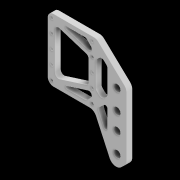
# Autodesk Inventor part: UpperShoulderBracket
Saved by Autodesk Inventor 2020 (Build 240168000, 168)
## iProperties
Created: 2020-04-26
Part Number: UpperShoulderBracket
Material: Generic
Document SubType Name: Sheet Metal
Designer: valer
Density: 1 g/cm^3
Sheet Metal Rule: Default
Appearance: Default
Author: valer
Autodesk Inventor part; units mm, degrees
ref_plane "YZ Plane" through (0, 0, 0) normal (1, 0, 0) x (0, 1, 0)
ref_plane "XZ Plane" through (0, 0, 0) normal (0, 1, 0) x (-1, 0, 0)
ref_plane "XY Plane" through (0, 0, 0) normal (0, 0, 1) x (1, 0, 0)
sketch "Sketch1" plane through (0, 0, 0) normal (0, 0, 1) x (1, 0, 0)
  line L0 (-42.4511, 36.83) -> (-26.4283, 36.83)
  arc A0 (-24.6322, 36.0861) -> (-26.4283, 36.83) centre (-26.4283, 34.29) ccw
  line L1 (-24.6322, 36.0861) -> (-21.0157, 32.4696)
  arc A1 (-23.5785, 28.252) -> (-21.0157, 32.4696) centre (-22.8118, 30.6735) ccw
  line L2 (-23.5785, 28.252) -> (-42.8345, 34.3492)
  arc A2 (-42.4511, 36.83) -> (-42.8345, 34.3492) centre (-42.4511, 35.56) ccw
  line L3 (-42.8345, -8.9492) -> (-23.5785, -2.852)
  arc A3 (-21.0157, -7.0696) -> (-23.5785, -2.852) centre (-22.8118, -5.2735) ccw
  line L4 (-21.0157, -7.0696) -> (-24.6322, -10.6861)
  arc A4 (-26.4283, -11.43) -> (-24.6322, -10.6861) centre (-26.4283, -8.89) ccw
  line L5 (-26.4283, -11.43) -> (-42.4511, -11.43)
  arc A5 (-42.8345, -8.9492) -> (-42.4511, -11.43) centre (-42.4511, -10.16) ccw
  line L6 (-52.9416, -3.8174) -> (-52.9416, 29.2174)
  arc A6 (-48.8082, 32.2443) -> (-52.9416, 29.2174) centre (-49.7666, 29.2174) ccw
  line L7 (-48.8082, 32.2443) -> (-25.2598, 24.7879)
  arc A7 (-23.0433, 21.7611) -> (-25.2598, 24.7879) centre (-26.2183, 21.7611) ccw
  line L8 (-23.0433, 21.7611) -> (-23.0433, 3.6389)
  arc A8 (-25.2598, 0.6121) -> (-23.0433, 3.6389) centre (-26.2183, 3.6389) ccw
  line L9 (-25.2598, 0.6121) -> (-48.8082, -6.8443)
  arc A9 (-52.9416, -3.8174) -> (-48.8082, -6.8443) centre (-49.7666, -3.8174) ccw
  line L10 (-6.35, 22.8627) -> (-6.35, 2.5373)
  arc A10 (-7.3432, 0.2307) -> (-6.35, 2.5373) centre (-9.525, 2.5373) ccw
  line L11 (-7.3432, 0.2307) -> (-9.3482, -1.6658)
  arc A11 (-13.775, -1.6043) -> (-9.3482, -1.6658) centre (-11.53, 0.6408) ccw
  line L12 (-13.775, -1.6043) -> (-15.7633, 0.384)
  arc A12 (-16.6933, 2.629) -> (-15.7633, 0.384) centre (-13.5183, 2.629) ccw
  line L13 (-16.6933, 2.629) -> (-16.6933, 22.771)
  arc A13 (-15.7633, 25.016) -> (-16.6933, 22.771) centre (-13.5183, 22.771) ccw
  line L14 (-15.7633, 25.016) -> (-13.775, 27.0043)
  arc A14 (-9.3482, 27.0658) -> (-13.775, 27.0043) centre (-11.53, 24.7592) ccw
  line L15 (-9.3482, 27.0658) -> (-7.3432, 25.1693)
  arc A15 (-6.35, 22.8627) -> (-7.3432, 25.1693) centre (-9.525, 22.8627) ccw
  circle A16 centre (-55.8683, 24.7103) radius 1.27
  circle A17 centre (-55.8683, 0.7103) radius 1.27
  circle A18 centre (-19.8683, -11.2897) radius 1.27
  circle A19 centre (-19.8683, 12.7103) radius 1.27
  circle A20 centre (-19.8683, 36.7103) radius 1.27
  circle A21 centre (-19.8683, 24.7103) radius 1.27
  circle A22 centre (-19.8683, 0.7103) radius 1.27
  circle A23 centre (-55.8683, -11.2897) radius 1.27
  circle A24 centre (-55.8683, 12.7103) radius 1.27
  circle A25 centre (-55.8683, 36.7103) radius 1.27
  arc A26 (-54.2116, 40.64) -> (-59.2916, 35.56) centre (-54.2116, 35.56) ccw
  line L16 (-59.2916, -10.16) -> (-59.2916, 35.56)
  arc A27 (-59.2916, -10.16) -> (-54.2116, -15.24) centre (-54.2116, -10.16) ccw
  line L17 (-18.1336, -15.24) -> (-54.2116, -15.24)
  line L18 (0, 0) -> (0, 25.4) construction
  line L19 (-14.6427, 39.2505) -> (0, 25.4)
  arc A28 (-14.6427, 39.2505) -> (-18.1336, 40.64) centre (-18.1336, 35.56) ccw
  line L20 (-54.2116, 40.64) -> (-18.1336, 40.64)
  line L21 (0, 25.4) -> (10.5833, 15.3892)
  line L22 (10.5833, 15.3892) -> (10.5833, -42.7021)
  circle A29 centre (2.1167, 11.7435) radius 3.175
  line L23 (2.1167, 11.7435) -> (2.1167, -39.0565) construction
  circle A30 centre (2.1167, -39.0565) radius 3.175
  line L24 (-0.6484, -53.3263) -> (10.5833, -42.7021)
  line L25 (-18.1336, -15.24) -> (-0.6484, -53.3263)
  circle A31 centre (2.1167, -6.0365) radius 3.175
  circle A32 centre (2.1167, -21.2765) radius 3.175
  dimension "d0" = 8.4667
  dimension "d1" = 8.4667
  dimension "d2" = 8.4667
  dimension "d6" = 8.4667
  dimension "d7" = 6.35
  dimension "d10" = 50.8
  dimension "d11" = 8.4667
  dimension "d12" = 17.78
  dimension "d13" = 17.78
  measures "d0" distance from line of L10 L23.start
  measures "d1" distance from line of L22 L23.start
  measures "d2" distance from line of L21 L23.start
  measures "d6" distance from line of L25 L23.end
  measures "d7" diameter of A29
  measures "d10" distance of L23.start L23.end
  measures "d11" distance from line of L24 A30.centre
  measures "d12" distance of A31.centre L23.start
  measures "d13" distance of L23.end A32.centre
extrude "Plate2" add sketch "Sketch1" along normal blind 5.08
fillet "Fillet1" radius 6.35 4 edges at (-18.1336, -15.24, 2.54) (-0.6484, -53.3263, 2.54) (10.5833, -42.7021, 2.54) (10.5833, 15.3892, 2.54)
sketch "Sketch2" plane through (0, 0, 5.08) normal (0, 0, 1) x (1, 0, 0)
  line L0 (-6.35, -4.0743) -> (-15.2168, -12.4614)
  line L1 (-15.2168, -12.4614) -> (-6.35, -31.7753)
  line L2 (-6.35, -31.7753) -> (-6.35, -4.0743)
  line L3 (-6.35, 22.8627) -> (-6.35, 2.5373) projected
  line L4 (-22.2055, -15.24) -> (-54.2116, -15.24) projected
  line L5 (-26.4283, -11.43) -> (-42.4511, -11.43) projected
  line L6 (-4.3455, -45.2733) -> (-16.4346, -18.9406) projected
  line L7 (-7.3432, 0.2307) -> (-9.3482, -1.6658) projected
  point P0 (0, 0)
  dimension "d15" = 3.81
  dimension "d16" = 3.81
  dimension "d17" = 3.81
  constraints: 6 end point, 2 parallel, 1 collinear
  measures "d15" distance between parallel lines of L4 L5
  measures "d16" distance between parallel lines of L6 L1
  measures "d17" distance between parallel lines of L7 L0
extrude "Extrusion1" cut sketch "Sketch2" against normal blind 25.4
fillet "Fillet2" radius 1.778 2 edges at (-6.35, -31.7753, 2.54) (-6.35, -4.0743, 2.54)
fillet "Fillet3" radius 2.54 1 edges at (-15.2168, -12.4614, 2.54)
equation "\"d14\" = Thickness"
equation "\"BendRadius\" = Thickness"
equation "\"BendReliefWidth\" = Thickness"
equation "\"BendReliefDepth\" = 0.5 * Thickness"
equation "\"CornerReliefSize\" = 4 * Thickness"
equation "\"MinimumRemnant\" = 2 * Thickness"
equation "\"TransitionRadius\" = BendRadius"
equation "\"JacobiRadiusSize\" = BendRadius"
equation "\"GapSize\" = Thickness"
equation "\"Thickness\" = 5.08"
body "Solid1"
body "Solid2"
